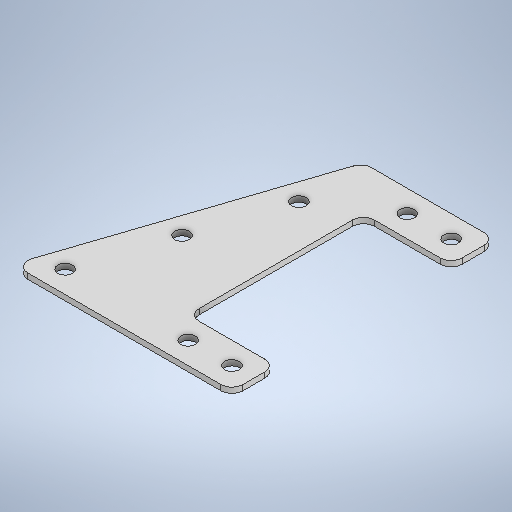
# Autodesk Inventor part: Intake Funnel
Saved by Autodesk Inventor 2025.2 (Build 292293000, 293)
## iProperties
Created: 2024-11-27
Part Number: Intake Funnel
Material: Generic
Document SubType Name: Modeling
Designer: jerem
Density: 1 g/cm^3
Appearance: Default
Author: jerem
Autodesk Inventor part; units mm, degrees
ref_plane "YZ Plane" through (0, 0, 0) normal (1, 0, 0) x (0, 1, 0)
ref_plane "XZ Plane" through (0, 0, 0) normal (0, 1, 0) x (-1, 0, 0)
ref_plane "XY Plane" through (0, 0, 0) normal (0, 0, 1) x (1, 0, 0)
sketch "Sketch1" plane through (0, 0, 0) normal (0, 1, 0) x (-1, 0, 0)
  line L0 (0, -3.175) -> (0, -9.525)
  line L1 (3.175, -12.7) -> (22.225, -12.7)
  line L2 (25.4, -15.875) -> (25.4, -60.325)
  line L3 (22.225, -63.5) -> (3.175, -63.5)
  line L4 (0, -66.675) -> (0, -73.025)
  line L5 (3.175, -76.2) -> (35.8116, -76.2)
  line L6 (38.8237, -74.029) -> (62.107, -4.179)
  line L7 (59.0949, 0) -> (3.175, 0)
  circle A0 centre (6.35, -6.35) radius 2.1209
  circle A1 centre (19.05, -6.35) radius 2.1209
  circle A2 centre (19.05, -69.85) radius 2.1209
  circle A3 centre (6.35, -69.85) radius 2.1209
  circle A4 centre (54.6898, -6.35) radius 2.1209
  circle A5 centre (46.2232, -31.75) radius 2.1209
  circle A6 centre (37.7565, -57.15) radius 2.1209
  arc A7 (62.107, -4.179) -> (59.0949, 0) centre (59.0949, -3.175) ccw
  arc A8 (3.175, 0) -> (0, -3.175) centre (3.175, -3.175) ccw
  arc A9 (0, -9.525) -> (3.175, -12.7) centre (3.175, -9.525) ccw
  arc A10 (22.225, -63.5) -> (25.4, -60.325) centre (22.225, -60.325) ccw
  arc A11 (25.4, -15.875) -> (22.225, -12.7) centre (22.225, -15.875) ccw
  arc A12 (3.175, -63.5) -> (0, -66.675) centre (3.175, -66.675) ccw
  arc A13 (0, -73.025) -> (3.175, -76.2) centre (3.175, -73.025) ccw
  arc A14 (35.8116, -76.2) -> (38.8237, -74.029) centre (35.8116, -73.025) ccw
  point P0 (0, 0)
  point P1 (0, -12.7)
  point P2 (25.4, -63.5)
  point P3 (0, -63.5)
  point P4 (0, -76.2)
  point P5 (38.1, -76.2)
  point P6 (63.5, 0)
  dimension "d0" = 63.5
  dimension "d1" = 76.2
  dimension "d2" = 12.7
  dimension "d3" = 12.7
  dimension "d4" = 25.4
  dimension "d5" = 38.1
  dimension "d6" = 4.2418
  dimension "d7" = 6.35
  dimension "d8" = 6.35
  dimension "d9" = 12.7
  dimension "d10" = 6.35
  dimension "d11" = 6.35
  dimension "d12" = 6.35
  dimension "d13" = 12.7
  dimension "d14" = 6.35
  dimension "d15" = 6.35
  dimension "d16" = 6.35
  dimension "d17" = 6.35
  dimension "d18" = 6.35
  dimension "d19" = 25.4
  dimension "d20" = 25.4
  dimension "d21" = 3.175
  constraints: 16 end point, 16 point on circle, 16 point on line, 16 tangent, 15 centre point, 13 equal radius, 5 perpendicular, 1 vertical
  measures "d0" distance of point (63.5, 0) point (0, 0)
  measures "d1" distance between parallel lines of L5 L7
  measures "d2" distance of point (0, 0) point (0, -12.7)
  measures "d3" distance of point (0, -63.5) point (0, -76.2)
  measures "d4" distance of point (25.4, -63.5) point (0, -63.5)
  measures "d5" distance of point (0, -76.2) point (38.1, -76.2)
  measures "d6" diameter of A0
  measures "d7" distance from line of L0 A0.centre
  measures "d8" distance from line of L1 A0.centre
  measures "d9" distance of A0.centre A1.centre
  measures "d10" distance from line of L1 A1.centre
  measures "d11" distance from line of L4 A3.centre
  measures "d12" distance from line of L3 A3.centre
  measures "d13" distance of A3.centre A2.centre
  measures "d14" distance from line of L5 A2.centre
  measures "d15" distance from line of L6 A6.centre
  measures "d16" distance from line of L6 A5.centre
  measures "d17" distance from line of L6 A4.centre
  measures "d18" distance from line of L7 A4.centre
  measures "d19" vertical distance of A4.centre A5.centre
  measures "d20" vertical distance of A5.centre A6.centre
  measures "d21" radius of A7
extrude "Extrusion1" add sketch "Sketch1" along normal blind 1.5875
body "Solid1"
